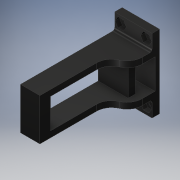
# Autodesk Inventor part: SupportServo
Saved by Autodesk Inventor 2019 (Build 230136000, 136)
## iProperties
Created: 2019-07-30
Part Number: SupportServo
Material: Plastique ABS
Document SubType Name: Modeling
Designer: Sébastien DI MERCURIO
Mass: 88.298 g
Surface Area: 125.14 cm^2
Volume: 83.3 cm^3
Density: 1.06 g/cm^3
Appearance: Lustré - Noir
Author: Sébastien DI MERCURIO
Autodesk Inventor part; units mm, degrees
ref_plane "YZ Plane" through (0, 0, 0) normal (1, 0, 0) x (0, 1, 0)
ref_plane "XZ Plane" through (0, 0, 0) normal (0, 1, 0) x (-1, 0, 0)
ref_plane "XY Plane" through (0, 0, 0) normal (0, 0, 1) x (1, 0, 0)
sketch "Esquisse1" plane through (0, 0, 0) normal (0, 0, 1) x (1, 0, 0)
  line L0 (0, 0) -> (25, 0)
  line L1 (25, 0) -> (25, 49)
  line L2 (25, 49) -> (0, 49)
  line L3 (0, 49) -> (0, 0)
  dimension "d0" = 25
  dimension "d1" = 49
  constraints: 8 end point, 2 parallel, 1 horizontal, 1 perpendicular
  measures "d0" distance of L0.start L0.end
  measures "d1" distance between parallel lines of L0 L2
extrude "Extrusion1" add sketch "Esquisse1" along normal blind 68
sketch "Esquisse2" plane through (0, 0, 68) normal (0, 0, 1) x (1, 0, 0)
  line L0 (0, 49) -> (0, 0) projected
  line L1 (25, 0) -> (25, 49) projected
  line L2 (0, 0) -> (25, 0)
  line L3 (25, 0) -> (25, 10.5)
  line L4 (25, 10.5) -> (0, 10.5)
  line L5 (0, 10.5) -> (0, 0)
  line L6 (0, 49) -> (25, 49)
  line L7 (25, 49) -> (25, 38.5)
  line L8 (25, 38.5) -> (0, 38.5)
  line L9 (0, 38.5) -> (0, 49)
  dimension "d4" = 49
  dimension "d5" = 28
  dimension "d6" = 10.5
  constraints: 16 end point, 4 parallel, 3 point on line, 2 horizontal, 2 perpendicular
  measures "d4" distance of L0.start L0.end
  measures "d5" distance of L8.end L4.end
  measures "d6" distance of L4.end L0.end
extrude "Extrusion2" cut sketch "Esquisse2" against normal blind 63 contours L6 L1 L8 L0 | L4 L1 L2 L0
sketch "Esquisse3" plane through (0, 0, 68) normal (0, 0, 1) x (1, 0, 0)
  line L0 (25, 38.5) -> (0, 38.5) projected
  line L1 (25, 10.5) -> (13, 10.5)
  line L2 (13, 10.5) -> (13, 38.5)
  line L3 (13, 38.5) -> (25, 38.5)
  line L4 (25, 38.5) -> (25, 10.5)
  line L5 (0, 38.5) -> (0, 10.5) projected
  point P0 (0, 0)
  dimension "d9" = 13
  constraints: 8 end point, 2 parallel, 1 horizontal, 1 perpendicular, 1 point on line
  measures "d9" distance between parallel lines of L5 L2
extrude "Extrusion3" cut sketch "Esquisse3" against normal blind 48
sketch "Esquisse4" plane through (25, 0, 0) normal (1, 0, 0) x (0, 0, -1)
  line L0 (-3, 14.5) -> (-61, 14.5)
  line L1 (-61, 14.5) -> (-61, 34.5)
  line L2 (-61, 34.5) -> (-3, 34.5)
  line L3 (-3, 34.5) -> (-3, 14.5)
  line L4 (-68, 10.5) -> (-68, 38.5) projected
  line L5 (-20, 10.5) -> (-68, 10.5) projected
  point P0 (0, 0)
  dimension "d12" = 58
  dimension "d13" = 7
  dimension "d14" = 28
  dimension "d15" = 20
  dimension "d16" = 4
  constraints: 8 end point, 2 parallel, 1 horizontal, 1 perpendicular
  measures "d12" distance of L0.start L0.end
  measures "d13" distance between parallel lines of L4 L1
  measures "d14" distance of L4.end L4.start
  measures "d15" distance of L1.end L0.end
  measures "d16" distance between parallel lines of L0 L5
extrude "Extrusion4" cut sketch "Esquisse4" against normal through all
sketch "Esquisse5" plane through (0, 0, 5) normal (0, 0, 1) x (1, 0, 0)
  circle A0 centre (21, 44) radius 1.5
  circle A1 centre (4, 44) radius 1.5
  circle A2 centre (4, 5) radius 1.5
  circle A3 centre (21, 5) radius 1.5
  line L0 (0, 38.5) -> (0, 49) projected
  line L1 (25, 49) -> (25, 38.5) projected
  line L2 (25, 0) -> (0, 0) projected
  line L3 (0, 49) -> (25, 49) projected
  dimension "d19" = 39
  dimension "d20" = 17
  dimension "d21" = 3
  dimension "d22" = 25
  dimension "d23" = 4
  dimension "d24" = 49
  dimension "d25" = 5
  constraints: 4 centre point, 3 equal radius, 2 horizontal alignment, 2 vertical alignment
  measures "d19" distance of A3.centre A0.centre
  measures "d20" distance of A1.centre A0.centre
  measures "d21" diameter of A0
  measures "d22" distance between parallel lines of L0 L1
  measures "d23" distance from line of L1 A0.centre
  measures "d24" distance between parallel lines of L2 L3
  measures "d25" distance from line of L3 A0.centre
extrude "Extrusion5" cut sketch "Esquisse5" against normal through all
sketch "Esquisse6" plane through (0, 0, 5) normal (0, 0, 1) x (1, 0, 0)
  circle A0 centre (21, 44) radius 1.5 projected
  line L0 (24.7528, 44) -> (22.8764, 40.75)
  line L1 (22.8764, 40.75) -> (19.1236, 40.75)
  line L2 (19.1236, 40.75) -> (17.2472, 44)
  line L3 (17.2472, 44) -> (19.1236, 47.25)
  line L4 (19.1236, 47.25) -> (22.8764, 47.25)
  line L5 (22.8764, 47.25) -> (24.7528, 44)
  circle A1 centre (4, 44) radius 1.5 projected
  line L6 (7.7528, 44) -> (5.8764, 40.75)
  line L7 (5.8764, 40.75) -> (2.1236, 40.75)
  line L8 (2.1236, 40.75) -> (0.2472, 44)
  line L9 (0.2472, 44) -> (2.1236, 47.25)
  line L10 (2.1236, 47.25) -> (5.8764, 47.25)
  line L11 (5.8764, 47.25) -> (7.7528, 44)
  circle A2 centre (4, 5) radius 1.5 projected
  line L12 (7.7528, 5) -> (5.8764, 1.75)
  line L13 (5.8764, 1.75) -> (2.1236, 1.75)
  line L14 (2.1236, 1.75) -> (0.2472, 5)
  line L15 (0.2472, 5) -> (2.1236, 8.25)
  line L16 (2.1236, 8.25) -> (5.8764, 8.25)
  line L17 (5.8764, 8.25) -> (7.7528, 5)
  circle A3 centre (21, 5) radius 1.5 projected
  line L18 (24.7528, 5) -> (22.8764, 1.75)
  line L19 (22.8764, 1.75) -> (19.1236, 1.75)
  line L20 (19.1236, 1.75) -> (17.2472, 5)
  line L21 (17.2472, 5) -> (19.1236, 8.25)
  line L22 (19.1236, 8.25) -> (22.8764, 8.25)
  line L23 (22.8764, 8.25) -> (24.7528, 5)
  point P0 (0, 0)
  dimension "d28" = 6.5
  constraints: 48 end point, 4 coincident, 4 horizontal alignment, 3 parallel, 52 other
  measures "d28" distance between parallel lines of L20 L23
extrude "Extrusion6" cut sketch "Esquisse6" against normal blind 3
fillet "Congé1" radius 10 4 edges at (25, 36.5, 20) (13, 36.5, 20) (13, 12.5, 20) (25, 12.5, 20)
fillet "Congé2" radius 1.5 2 edges at (12.5, 38.5, 5) (12.5, 10.5, 5)
sketch "Esquisse7" plane through (0, 0, 0) normal (-1, 0, 0) x (0, 0, 1)
  line L0 (3, 34.5) -> (61, 34.5) projected
  line L1 (16, 34.5) -> (11, 34.5)
  line L2 (11, 34.5) -> (11, 14.5)
  line L3 (11, 14.5) -> (16, 14.5)
  line L4 (16, 14.5) -> (16, 34.5)
  line L5 (61, 14.5) -> (3, 14.5) projected
  line L6 (3, 14.5) -> (3, 34.5) projected
  line L7 (61, 34.5) -> (61, 14.5) projected
  point P0 (0, 0)
  dimension "d33" = 5
  dimension "d45" = 45
  constraints: 8 end point, 2 parallel, 1 collinear, 1 horizontal, 1 perpendicular, 1 point on line
  measures "d33" distance between parallel lines of L2 L4
  measures "d45" distance between parallel lines of L4 L7
extrude "Extrusion7" add sketch "Esquisse7" against normal blind 20 contours L0 L4 L3 L2
sketch "Esquisse8" plane through (0, 0, 0) normal (-1, 0, 0) x (0, 0, 1)
  circle A0 centre (63, 29.5) radius 1.25
  circle A1 centre (63, 19.5) radius 1.25
  circle A2 centre (14.4, 29.5) radius 1.25
  circle A3 centre (14.4, 19.5) radius 1.25
  line L0 (6.5, 10.5) -> (68, 10.5) projected
  line L1 (68, 38.5) -> (6.5, 38.5) projected
  line L2 (68, 38.5) -> (68, 10.5) projected
  point P0 (0, 0)
  dimension "d37" = 2.5
  dimension "d38" = 10
  dimension "d39" = 28
  dimension "d40" = 9
  dimension "d41" = 48.6
  dimension "d42" = 5
  constraints: 4 centre point, 3 equal radius, 2 horizontal alignment, 2 vertical alignment
  measures "d37" diameter of A0
  measures "d38" distance of A1.centre A0.centre
  measures "d39" distance between parallel lines of L0 L1
  measures "d40" distance from line of L1 A0.centre
  measures "d41" distance of A2.centre A0.centre
  measures "d42" distance from line of L2 A0.centre
extrude "Extrusion8" cut sketch "Esquisse8" against normal blind 7
equation "\"d6\" = -0.5 * d5 + 0.5 * d4"
equation "\"d16\" = -0.5 * d15 + 0.5 * d14"
equation "\"d23\" = -0.5 * d20 + 0.5 * d22"
equation "\"d25\" = -0.5 * d19 + 0.5 * d24"
equation "\"d40\" = -0.5 * d38 + 0.5 * d39"
